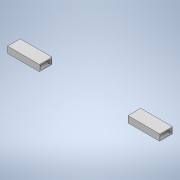
# Autodesk Inventor part: Intake - 2 by 1 Aluminum Mounting CrossBar
Saved by Autodesk Inventor 2020 (Build 240168000, 168)
## iProperties
Created: 2020-02-05
Part Number: Intake - 2 by 1 Aluminum Mounting CrossBar
Material: Generic
Document SubType Name: Modeling
Designer: aidan
Density: 1 g/cm^3
Appearance: Default
Author: aidan
Autodesk Inventor part; units mm, degrees
ref_plane "YZ Plane" through (0, 0, 0) normal (1, 0, 0) x (0, 1, 0)
sketch "Sketch1" plane through (0, 0, 0) normal (1, 0, 0) x (0, 1, 0)
  line L0 (0, 0) -> (25.4, 0)
  line L1 (25.4, 0) -> (25.4, -50.8)
  line L2 (25.4, -50.8) -> (0, -50.8)
  line L3 (0, -50.8) -> (0, 0)
  line L4 (22.225, -3.175) -> (3.175, -3.175)
  line L5 (3.175, -3.175) -> (3.175, -47.625)
  line L6 (3.175, -47.625) -> (22.225, -47.625)
  line L7 (22.225, -47.625) -> (22.225, -3.175)
  dimension "d0" = 25.4
  dimension "d1" = 50.8
  dimension "d2" = 3.175
  dimension "d3" = 3.175
  dimension "d4" = 3.175
  dimension "d5" = 3.175
  constraints: 16 end point, 4 parallel, 2 horizontal, 2 perpendicular
  measures "d0" distance of L1.end L2.end
  measures "d1" distance of L0.end L1.end
  measures "d2" distance between parallel lines of L2 L6
  measures "d3" distance between parallel lines of L1 L7
  measures "d4" distance between parallel lines of L0 L4
  measures "d5" distance between parallel lines of L3 L5
extrude "Extrusion1" add sketch "Sketch1" along normal blind 127
sketch "Sketch2" plane through (0, 25.4, 0) normal (0, 1, 0) x (1, 0, 0)
  line L0 (6.35, 6.35) -> (19.05, 6.35)
  line L1 (19.05, 6.35) -> (19.05, 44.45)
  line L2 (19.05, 44.45) -> (6.35, 44.45)
  line L3 (6.35, 44.45) -> (6.35, 6.35)
  line L4 (0, 50.8) -> (0, 0) projected
  line L5 (0, 0) -> (127, 0) projected
  dimension "d8" = 12.7
  dimension "d9" = 38.1
  dimension "d10" = 6.35
  dimension "d11" = 6.35
  constraints: 8 end point, 2 parallel, 1 horizontal, 1 perpendicular
  measures "d8" distance of L2.end L1.end
  measures "d9" distance of L1.end L0.end
  measures "d10" distance between parallel lines of L4 L3
  measures "d11" distance between parallel lines of L5 L0
sketch "Sketch3" plane through (0, 3.175, -3.175) normal (0, 1, 0) x (1, 0, 0)
  line L0 (0, 47.625) -> (127, 47.625) projected
  line L1 (19.05, 41.275) -> (6.35, 41.275) projected
  line L2 (19.05, 3.175) -> (19.05, 41.275) projected
  line L3 (6.35, 41.275) -> (6.35, 3.175) projected
  line L4 (6.35, 3.175) -> (19.05, 3.175) projected
  point P0 (0, -3.175)
hole "Hole1" at (19.05, 3.175, -44.45) at (6.35, 3.175, -44.45) at (19.05, 3.175, -6.35) at (6.35, 3.175, -6.35) direction (0, -1, 0) diameter 3.175 end through all
ref_plane "Work Plane1" through (63.5, 0, 0) normal (-1, 0, 0) x (0, 0, 1)
mirror "Mirror1" about plane through (63.5, 0, 0) normal (-1, 0, 0) of "Hole1"
ref_plane "Work Plane2" through (-177.8, 0, 0) normal (-1, 0, 0) x (0, 0, 1)
mirror "Mirror2" about plane through (-177.8, 0, 0) normal (-1, 0, 0)
body "Solid1"
